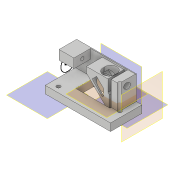
# Autodesk Inventor part: cellSTORM_dichroic_mirror_adjuster_tmp
Saved by Autodesk Inventor 2019.4 (Build 234330000, 330)
## iProperties
Created: 2020-06-30
Part Number: cellSTORM_dichroic_mirror_adjuster_tmp
Material: Generic
Document SubType Name: Modeling
Designer: diederichbenedict
Density: 1 g/cm^3
Appearance: Default
Author: diederichbenedict
Autodesk Inventor part; units mm, degrees
ref_plane "YZ Plane" through (0, 0, 0) normal (1, 0, 0) x (0, 1, 0)
ref_plane "XZ Plane" through (0, 0, 0) normal (0, 1, 0) x (-1, 0, 0)
ref_plane "XY Plane" through (0, 0, 0) normal (0, 0, 1) x (1, 0, 0)
ref_plane "Work Plane1" through (-9.4272, 11.5884, 0.05) normal (0, 0, 1) x (1, 0, 0)
sketch "Sketch1" plane through (-9.4272, 11.5884, 0.05) normal (0, 0, 1) x (1, 0, 0)
  line L0 (-5.9698, 7.5884) -> (-5.9698, -7.5884) projected
  line L1 (-5.9698, -7.5884) -> (5.9698, -7.5884) projected
  line L2 (5.9698, -7.5884) -> (5.9698, 7.5884) projected
  line L3 (5.9698, 7.5884) -> (-5.9698, 7.5884) projected
  line L4 (-6.0698, 7.6884) -> (-6.0698, -7.6884)
  line L5 (-6.0698, -7.6884) -> (6.0698, -7.6884)
  line L6 (6.0698, -7.6884) -> (6.0698, 7.6884)
  line L7 (6.0698, 7.6884) -> (-6.0698, 7.6884)
  line L8 (-6.0698, -7.6884) -> (-21.0698, -7.6884)
  line L9 (-21.0698, -7.6884) -> (-21.0698, 9.3116)
  line L10 (6.0698, -7.6884) -> (11.0698, -7.6884)
  line L11 (11.0698, -7.6884) -> (11.0698, 9.3116)
  line L12 (11.0698, 9.3116) -> (-21.0698, 9.3116)
  point P0 (9.4272, -11.5884)
  dimension "d0" = 0.1
  dimension "d1" = 15
  dimension "d2" = 17
  dimension "d3" = 5
  dimension "d4" = 90
  constraints: 18 end point, 4 point on line, 2 horizontal, 2 perpendicular, 3 other
  measures "d0" distance between parallel lines of L3 L7
  measures "d1" distance of L8.start L8.end
  measures "d2" distance of L8.end L9.end
  measures "d3" distance of L10.start L10.end
  measures "d4" angle of L11 L10
extrude "Extrusion1" add sketch "Sketch1" along normal blind 0.5 contours L3 L2 L1 L0 | L7 L6 L5 L4 | L4 L8 L9 L12 L11 L10 L6 L7
sketch "Sketch3" plane through (-9.4272, 11.5884, 0.55) normal (0, 0, 1) x (1, 0, 0)
  line L0 (-2.9698, 4.4671) -> (-0.8485, 6.5884) projected
  line L1 (2.2627, -0.7655) -> (-2.9698, 4.4671) projected
  line L2 (2.8284, -0.1998) -> (2.2627, -0.7655) projected
  line L3 (2.8284, 2.9115) -> (2.8284, -0.1998) projected
  line L4 (-0.8485, 6.5884) -> (2.8284, 2.9115) projected
  line L5 (5.3213, 2.5399) -> (6.0698, 1.7914)
  line L6 (6.0698, 1.7914) -> (6.0698, -4.8892)
  line L7 (6.0698, 7.6884) -> (6.0698, -7.5884) projected
  line L8 (6.0698, -4.8892) -> (5.1675, -5.7915)
  line L9 (5.1675, -5.7915) -> (-5.0912, 4.4671)
  line L10 (3.0284, 2.9943) -> (3.0284, -0.2826)
  line L11 (3.0284, -0.2826) -> (2.2627, -1.0483)
  line L12 (2.2627, -1.0483) -> (-3.2527, 4.4671)
  line L13 (-3.2527, 4.4671) -> (-0.8485, 6.8713)
  line L14 (-0.8485, 6.8713) -> (3.0284, 2.9943)
  line L15 (6.0698, -4.8892) -> (7.0698, -4.8892)
  line L16 (7.0698, -4.8892) -> (7.0698, -4.3892)
  line L17 (7.0698, -4.3892) -> (6.0698, -4.3892)
  line L18 (6.0698, -4.3892) -> (6.0698, -4.8892)
  line L19 (-11.0698, 9.4116) -> (11.0698, 9.4116) projected
  line L20 (-21.0698, -7.6884) -> (11.0698, -7.6884) projected
  line L21 (11.0698, 9.4116) -> (7.0698, 9.4116)
  line L22 (7.0698, 9.4116) -> (7.0698, -7.6884)
  line L23 (7.0698, -7.6884) -> (11.0698, -7.6884)
  line L24 (11.0698, -7.6884) -> (11.0698, 9.4116)
  line L25 (-5.0912, 4.4671) -> (-6.3481, 5.724)
  line L26 (-6.3481, 8.7553) -> (-0.8485, 8.7553)
  line L27 (-0.8485, 8.7553) -> (5.3213, 8.7553)
  line L28 (5.3213, 8.7553) -> (5.3213, 2.5399)
  line L29 (-5.0912, 4.4671) -> (-4.0305, 5.5278)
  line L30 (-1.9092, 7.6491) -> (-1.7678, 7.7905)
  line L31 (-6.3481, 5.724) -> (-6.3481, 5.724)
  line L32 (-6.3481, 5.724) -> (-6.3481, 8.7553)
  point P0 (9.4272, -11.5884)
  point P1 (11.0698, -7.6884)
  dimension "d10" = 1.5
  dimension "d11" = 1.5
  dimension "d14" = 0.2
  dimension "d15" = 1
  dimension "d16" = 0.5
  constraints: 50 end point, 11 parallel, 5 perpendicular, 5 point on line, 4 horizontal, 1 collinear, 1 vertical, 6 other
  measures "d10" distance between parallel lines of L9 L1
  measures "d11" distance between parallel lines of L5 L4
  measures "d14" distance between parallel lines of L4 L14
  measures "d15" distance of L17.end L16.end
  measures "d16" distance of L16.end L15.end
extrude "Extrusion3" add sketch "Sketch3" along normal blind 9 contours L5 L6 L8 L9 L25 L32 L26 L27 L28 | L17 L16 L15 L6 | L22 L19 L24 L20 L16
sketch "Sketch4" plane through (-30.497, 3.9, 0.55) normal (0, -1, 0) x (1, 0, 0)
  line L0 (26.2373, 0) -> (14.7218, 0) projected
  line L1 (26.2373, 0) -> (26.2373, 9) projected
  line L2 (14.7218, 9) -> (26.2373, 9) projected
  line L3 (28.1397, 0) -> (0, 0) projected
  line L4 (0, 0) -> (28.1397, 0)
  line L5 (28.1397, 0) -> (28.1397, 0.3)
  line L6 (28.1397, 0.3) -> (0, 0.3)
  line L7 (0, 0.3) -> (0, 0)
  line L8 (14.7218, 0) -> (14.7218, 9) projected
  point P0 (30.497, -0.55)
  point P1 (1.736, 0)
  point P2 (18.1397, 0)
  dimension "d41" = 0.3
  constraints: 8 end point, 2 parallel, 1 horizontal, 1 perpendicular
  measures "d41" distance between parallel lines of L3 L6
extrude "Extrusion4" cut sketch "Sketch4" against normal through all contours L0 L8 L6 L1 | L1 L6 L5 L3 | L3 L7 L6 L8
ref_plane "Work Plane3" through (1.6427, 4, -2.95) normal (1, 0, 0) x (0, 0, -1)
sketch "Sketch5" plane through (1.6427, 4, -2.95) normal (1, 0, 0) x (0, 0, -1)
  line L0 (-3, 16.9) -> (-3.5, 16.9) projected
  line L1 (-12.5, -0.1) -> (-12.5, 17) projected
  line L2 (-3, -0.1) -> (-12.5, -0.1) projected
  circle A0 centre (-8.4703, 13.9285) radius 1.4
  line L3 (-3, 16.9) -> (-3, -0.1) projected
  line L4 (-3.5, 17) -> (-3.5, 16.9) projected
  line L5 (-3.5, 17) -> (-12.5, 17) projected
  point P0 (-2.95, -4)
  dimension "d21" = 2.8
  constraints: 1 centre point
  measures "d21" diameter of A0
extrude "Extrusion5" cut sketch "Sketch5" against normal up to surface (5.7485 mm away) contours A0
sketch "Sketch6" plane through (-15.7753, 20.3438, 9.55) normal (0, 1, 0) x (1, 0, 0)
  circle A0 centre (8.3144, 3.85) radius 3.2
  line L0 (8.3144, 3.85) -> (8.3144, 4.8641) construction
  line L1 (11.5144, 3.85) -> (11.5144, 4.8641)
  line L2 (5.1144, 4.8641) -> (5.1144, 3.85)
  arc A1 (5.1144, 3.85) -> (11.5144, 3.85) centre (8.3144, 3.85) ccw
  arc A2 (11.5144, 4.8641) -> (5.1144, 4.8641) centre (8.3144, 4.8641) ccw
  point P0 (15.7753, 9.55)
  point P1 (8.3144, 4.3571)
  constraints: 8 end point, 4 point on circle, 4 tangent, 3 centre point, 1 concentric, 1 midpoint, 1 parallel, 1 vertical
extrude "Extrusion6" cut sketch "Sketch6" against normal through all
sketch "Sketch7" plane through (-30.497, 3.9, 0.55) normal (-1, 0, 0) x (0, 0, 1)
  circle A0 centre (4.4299, 8.2054) radius 3.6733
  point P0 (-0.55, -3.9)
  point P1 (5.45, 8.2054)
  constraints: 1 centre point
ref_plane "Work Plane2" through (-9.7807, 13.4392, 0.05) normal (-0.7071068, -0.7071068, 0) x (0, 0, 1)
sketch "Sketch8" plane through (-4.2597, 5.7969, 9.55) normal (-0.7071068, -0.7071068, 0) x (-0.7071068, 0.7071068, 0)
  line L0 (16.2855, 8.7) -> (0, 8.7) projected
  line L1 (0, 8.7) -> (0, 0) projected
  line L2 (16.2855, 0) -> (0, 0) projected
  ellipse E0 centre (4.5272, 3.85) end of major axis (9.0526, 3.85) minor radius 3.2 (0.0017, 3.85) -> (9.0526, 3.85) ccw projected
  ellipse E1 centre (4.5272, 4.8641) end of major axis (0.0017, 4.8641) minor radius 3.2 (9.0526, 4.8641) -> (0.0017, 4.8641) ccw projected
  line L3 (4.9374, 0.7098) -> (9.8018, 0.7098)
  line L4 (12.8018, 3.7098) -> (12.8018, 5.1494)
  line L5 (9.8018, 8.1494) -> (4.9374, 8.1494)
  line L6 (1.9374, 5.1494) -> (1.9374, 3.7098)
  arc A0 (9.8018, 0.7098) -> (12.8018, 3.7098) centre (9.8018, 3.7098) ccw
  arc A1 (12.8018, 5.1494) -> (9.8018, 8.1494) centre (9.8018, 5.1494) ccw
  arc A2 (4.9374, 8.1494) -> (1.9374, 5.1494) centre (4.9374, 5.1494) ccw
  arc A3 (1.9374, 3.7098) -> (4.9374, 0.7098) centre (4.9374, 3.7098) ccw
  line L7 (9.0526, 4.8641) -> (9.0526, 3.85) projected
  line L8 (16.2855, 8.7) -> (16.2855, 0) projected
  line L9 (0.0017, 3.85) -> (0.0017, 4.8641) projected
  point P0 (-7.1111, 9.55)
  dimension "d42" = 3
  constraints: 8 end point, 8 point on circle, 8 tangent, 4 centre point, 3 equal radius, 2 parallel, 1 horizontal, 1 perpendicular, 2 other
  measures "d42" radius of A0
extrude "Extrusion8" cut sketch "Sketch8" against normal up to surface (1.3 mm away) contours A2 L5 A1 L4 A0 L3 E0 L7 E1 | E1 L7 E0 L3 A3 L6 A2
ref_plane "Work Plane4" through (-9.4272, 11.5884, -2.95) normal (0, 0, -1) x (-1, 0, 0)
ref_plane "Work Plane7" through (-6.3987, 11.3058, 7.8996) normal (0, 1, 0) x (1, 0, 0)
ref_plane "Work Plane5" through (-3.3573, 3.9, 0.05) normal (0, -1, 0) x (1, 0, 0)
sketch "Sketch16" plane through (-3.3573, 3.9, 0.05) normal (0, -1, 0) x (1, 0, 0)
  line L0 (1, 0.5) -> (1, 9.5) projected
  line L1 (-27.1397, 0.5) -> (1, 0.5) projected
  line L2 (5, 0) -> (-27.1397, 0) projected
  line L3 (5, 0) -> (5, 9.5) projected
  line L4 (1, 9.5) -> (5, 9.5) projected
  line L5 (5, 0) -> (-27.1397, 0) projected
  line L6 (-12.1397, 0.5) -> (0, 0.5) projected
  line L7 (5, 0) -> (-27.1397, 0) projected
  line L8 (-27.1397, 0.5) -> (1, 0.5) projected
  line L9 (-27.1397, 0) -> (-27.1397, 0.5) projected
  line L10 (-12.1397, 0) -> (-12.1397, 0.5) projected
  circle A0 centre (5.0158, 8.95) radius 1 projected
  circle A1 centre (-16.4842, -6.55) radius 1 projected
  circle A2 centre (-22.9842, 13.95) radius 1 projected
  line L11 (-27.1287, 16.95) -> (8.0158, 16.95)
  line L12 (8.0158, 16.95) -> (8.0158, 0)
  line L13 (8.0158, 0) -> (-27.1287, 0)
  line L14 (-27.1287, 0) -> (-27.1287, 16.95)
  circle A3 centre (-22.9842, 13.95) radius 1
  circle A4 centre (5.0158, 8.95) radius 1
  line L15 (0.9985, 0.5) -> (-17.4842, 0.5)
  line L16 (-17.4842, 0.5) -> (-17.4842, 10.2078)
  line L17 (-17.4842, 10.2078) -> (0.9985, 10.2078)
  line L18 (0.9985, 10.2078) -> (0.9985, 0.5)
  line L19 (-27.1397, 0) -> (-27.1397, 0.5) projected
  point P0 (3.3573, -0.05)
  point P1 (0, 0)
  dimension "d53" = 3
  dimension "d54" = 3
  dimension "d55" = 2
  dimension "d56" = 2
  constraints: 16 end point, 4 parallel, 2 centre point, 2 coincident, 2 horizontal, 2 perpendicular, 1 point on line
  measures "d53" distance from line of A2.centre L11
  measures "d54" distance from line of L12 A0.centre
  measures "d55" diameter of A3
  measures "d56" diameter of A4
extrude "Extrusion15" add sketch "Sketch16" against normal blind 4 contours L18 L17 L16 L1 L14 L11 L12 L13 L3 A0 L4
ref_plane "Work Plane6" through (-29.3415, 3.9, 17) normal (0, -1, 0) x (1, 0, 0)
sketch "Sketch17" plane through (-29.3415, 3.9, 17) normal (0, -1, 0) x (1, 0, 0)
  arc A0 (30.9842, -8.9999) -> (30.1648, -7.45) centre (31, -8) ccw projected
  circle A1 centre (31, -8) radius 1
  point P0 (29.3415, -17)
  constraints: 1 centre point, 1 coincident, 1 concentric
extrude "Extrusion16" cut sketch "Sketch17" against normal through all
sketch "Sketch18" plane through (1.6427, 20.9, 0.55) normal (1, 0, 0) x (0, 0, -1)
  line L0 (0.5, 0) -> (0.5, -13) projected
  line L1 (0.5, 0) -> (0, 0) projected
  line L2 (0, 0.1) -> (0, 0) projected
  line L3 (0, 0.1) -> (-7.4501, 0.1) projected
  line L4 (-9, -6.7717) -> (-9, -0.5562) projected
  line L5 (-0.3, -6.7717) -> (-9, -6.7717) projected
  circle A0 centre (-4.1776, -3.2963) radius 1.45
  line L6 (-0.3, -0.5562) -> (-9, -0.5562) projected
  line L7 (-7.4501, 0.1) -> (-7.4501, -13) projected
  line L8 (-7.4501, -13) -> (0.5, -13) projected
  line L9 (-0.3, -6.7717) -> (-0.3, -0.5562) projected
  point P0 (0.55, -20.9)
  dimension "d61" = 2.9
  constraints: 1 centre point
  measures "d61" diameter of A0
extrude "Extrusion17" cut sketch "Sketch18" against normal up to surface (5.7485 mm away) contours A0
sketch "Sketch19" plane through (-9.4272, 11.5884, 9.55) normal (0, 0, 1) x (1, 0, 0)
  line L0 (7.0684, -4.8892) -> (7.0684, -4.3892) projected
  line L1 (7.0684, -4.3892) -> (6.0698, -4.3892) projected
  line L2 (6.0698, -4.3892) -> (6.0698, 1.7914) projected
  line L3 (6.0698, 1.7914) -> (5.3213, 2.5399) projected
  line L4 (5.3213, 2.5399) -> (5.3213, 8.7553) projected
  line L5 (5.3213, 8.7553) -> (-6.3481, 8.7553) projected
  line L6 (-6.3481, 8.7553) -> (-6.3481, 5.724) projected
  line L7 (-6.3481, 5.724) -> (5.1675, -5.7915) projected
  line L8 (5.1675, -5.7915) -> (6.0698, -4.8892) projected
  line L9 (6.0698, -4.8892) -> (7.0684, -4.8892) projected
  line L10 (3.0284, -0.2826) -> (2.2627, -1.0483) projected
  line L11 (2.2627, -1.0483) -> (-3.2527, 4.4671) projected
  line L12 (-3.2527, 4.4671) -> (-0.8485, 6.8713) projected
  line L13 (-0.8485, 6.8713) -> (3.0284, 2.9943) projected
  line L14 (3.0284, 2.9943) -> (3.0284, -0.2826) projected
  line L15 (2.2627, -1.0483) -> (-3.2527, 4.4671) projected
  line L16 (2.1513, -0.9369) -> (2.1513, -2.7754)
  line L17 (-6.3481, 5.724) -> (5.1675, -5.7915) projected
  line L18 (2.9122, 3.1105) -> (5.3213, 3.1105)
  line L19 (5.3213, 2.5399) -> (5.3213, 8.7553) projected
  line L20 (2.1513, -2.7754) -> (6.0698, -2.7754)
  point P0 (9.4272, -11.5884)
  constraints: 6 end point, 5 point on line, 1 parallel, 1 perpendicular, 1 vertical
extrude "Extrusion18" [suppressed]
sketch "Sketch20" plane through (-9.4272, 11.5884, 0.55) normal (0, 0, 1) x (1, 0, 0)
  line L0 (7.0684, -7.6884) -> (7.0684, -3.6884) projected
  line L1 (7.0684, -3.6884) -> (7.0698, -3.6884) projected
  line L2 (7.0698, -3.6884) -> (7.0698, 9.3116) projected
  line L3 (7.0698, 9.3116) -> (-21.0698, 9.3116) projected
  line L4 (-21.0698, 9.3116) -> (-21.0698, -7.6884) projected
  line L5 (-21.0698, -7.6884) -> (-21.0589, -7.6884) projected
  line L6 (-21.0589, -7.6884) -> (-21.0589, -3.6884) projected
  line L7 (-21.0589, -3.6884) -> (-11.4143, -3.6884) projected
  line L8 (-11.4143, -3.6884) -> (-11.4143, -7.6884) projected
  line L9 (-11.4143, -7.6884) -> (7.0684, -7.6884) projected
  line L10 (-21.0698, 9.3116) -> (-13.0698, 9.3116)
  line L11 (-13.0698, 9.3116) -> (-13.0698, 4.3116)
  line L12 (-13.0698, 4.3116) -> (-21.0698, 4.3116)
  line L13 (-21.0698, 4.3116) -> (-21.0698, 9.3116)
  point P0 (9.4272, -11.5884)
  dimension "d66" = 8
  dimension "d67" = 5
  constraints: 8 end point, 2 parallel, 1 horizontal, 1 perpendicular
  measures "d66" distance of L11.end L12.end
  measures "d67" distance of L10.end L11.end
extrude "Extrusion19" add sketch "Sketch20" along normal up to surface (9 mm away) contours L11 L12 L4 L3
sketch "Sketch21" plane through (-30.497, 3.9, 0.05) normal (-1, 0, 0) x (0, 0, 1)
  line L0 (0, 17) -> (9.5, 17) projected
  line L1 (0, 0) -> (0, 17) projected
  line L2 (0, 0) -> (0.5, 0) projected
  line L3 (0.5, 12) -> (0.5, 0) projected
  line L4 (0.5, 12) -> (9.5, 12) projected
  line L5 (9.5, 12) -> (9.5, 17) projected
  circle A0 centre (5, 14.5) radius 0.95
  point P0 (-0.05, -3.9)
  dimension "d70" = 1.9
  constraints: 1 centre point
  measures "d70" diameter of A0
extrude "Extrusion20" cut sketch "Sketch21" against normal up to surface (8 mm away) contours A0
body "Solid1"
